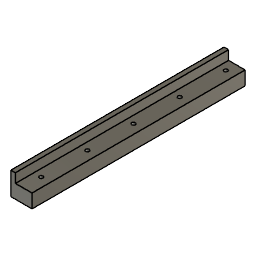
left engine cover part 2 (Autodesk Fusion 360 design; units mm, degrees)
Autodesk Fusion 360 part; units mm, degrees
sketch "Szkic1" plane through (0, 0, 0) normal (0, 0, 1) x (1, 0, 0)
  line L0 (29, -110) -> (29, -70)
  line L1 (-10, -75) -> (10, -75)
  line L2 (10, -75) -> (10, -98.8)
  line L3 (-45, -110) -> (29, -110)
  circle A0 centre (15, -80) radius 3.5
  circle A1 centre (15, -100) radius 3.5
  line L4 (-10, -98.8) -> (-10, -75)
  line L5 (10, -98.8) -> (-10, -98.8)
  circle A2 centre (-20, -100) radius 3.5
  circle A3 centre (-20, -80) radius 3.5
  line L6 (29, -70) -> (35, -70)
  line L7 (35, -70) -> (35, 160)
  circle A4 centre (25, -50) radius 1.75
  circle A5 centre (25, 0) radius 1.75
  circle A6 centre (25, 50) radius 1.75
  circle A7 centre (25, 100) radius 1.75
  line L8 (35, 160) -> (-45, 160)
  circle A8 centre (25, 150) radius 1.75
  circle A9 centre (-25, 150) radius 1.75
  line L9 (35, 160) -> (35, 135)
  line L10 (35, 135) -> (-45, 135)
  line L11 (-45, 135) -> (-45, 160)
  line L12 (-45, 160) -> (35, 160)
  line L13 (35, 135) -> (35, -70)
  line L14 (35, -70) -> (17, -70)
  line L15 (17, -70) -> (17, 135)
  line L16 (17, 135) -> (35, 135)
  line L17 (17, 135) -> (17, -70)
  line L18 (17, -70) -> (12, -70)
  line L19 (12, -70) -> (12, 135)
  line L20 (12, 135) -> (17, 135)
  dimension "d1" = 25
  dimension "d2" = 18
  dimension "d3" = 5
  constraint perpendicular L9 L10
  constraint parallel L9 L11
  constraint parallel L10 L12
  constraint coincident L7 L9.end
  constraint perpendicular L8 L9
  constraint perpendicular L13 L14
  constraint parallel L13 L15
  constraint parallel L14 L16
  constraint perpendicular L6 L13
  constraint perpendicular L17 L18
  constraint parallel L17 L19
  constraint parallel L18 L20
  measures "d1" distance of L7.end L9.end
  measures "d2" distance of L9.end L15.end
  measures "d3" distance of L15.end L19.end
extrude "Wyciągnięcie proste1" add sketch "Szkic1" along normal blind 15 contours L6 L7 L10 L13 L14 L15 L16 L17
extrude "Wyciągnięcie proste2" add sketch "Szkic1" along normal blind 25 contours L10 L15 L17 L18 L19 L20
extrude "Wyciągnięcie proste3" add 1 faces at (21.3333, 135, 5) along direction (0, 1, 0) blind 26
extrude "Wyciągnięcie proste4" cut sketch "Szkic1" along normal blind 27 contours A8
sketch "Szkic2" plane through (0, 0, 0) normal (0, 0, -1) x (1, 0, 0)
  circle A0 centre (25, -150) radius 1.75
  circle A1 centre (25, -50) radius 1.75
  circle A2 centre (25, -100) radius 1.75
  circle A3 centre (25, 0) radius 1.75
  circle A4 centre (25, 50) radius 1.75
  line L0 (35, -161) -> (35, 70)
  line L1 (35, 70) -> (12, 70)
  line L2 (12, 70) -> (12, -161)
  line L3 (12, -161) -> (35, -161)
  circle A5 centre (25, -150) radius 3.5
  circle A6 centre (25, -100) radius 2
  circle A7 centre (25, -50) radius 2
  circle A8 centre (25, 0) radius 2
  circle A9 centre (25, 50) radius 2
  dimension "d12" = 7
  dimension "d13" = 4
  dimension "d14" = 4
  dimension "d15" = 4
  dimension "d16" = 4
  constraint concentric A0 A5
  constraint concentric A2 A6
  constraint concentric A1 A7
  constraint concentric A3 A8
  constraint concentric A4 A9
  measures "d12" diameter of A5
  measures "d13" diameter of A6
  measures "d14" diameter of A7
  measures "d15" diameter of A8
  measures "d16" diameter of A9
extrude "Wyciągnięcie proste5" cut sketch "Szkic2" against normal blind 100 contours A6 | A7 | A8 | A9
extrude "Wyciągnięcie proste6" cut sketch "Szkic2" against normal blind 4 contours A5
sketch "Szkic3" plane through (0, 0, 0) normal (0, 0, -1) x (1, 0, 0)
  circle A0 centre (25, -150) radius 2
  dimension "d21" = 4
  measures "d21" diameter of A0
extrude "Wyciągnięcie proste7" cut sketch "Szkic3" against normal blind 100
